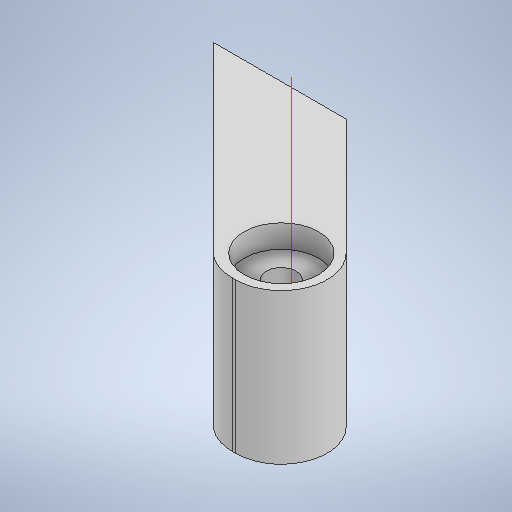
# Autodesk Inventor part: PingPongLauncherWinkel
Saved by Autodesk Inventor 2025 (Build 290162010, 162A)
## iProperties
Created: 2024-10-07
Part Number: PingPongLauncherWinkel
Material: Generisch
Document SubType Name: Modeling
Designer: max-h
Density: 1 g/cm^3
Appearance: Vorgabe
Author: max-h
Autodesk Inventor part; units mm, degrees
ref_plane "YZ Plane" through (0, 0, 0) normal (1, 0, 0) x (0, 1, 0)
ref_plane "XZ Plane" through (0, 0, 0) normal (0, 1, 0) x (-1, 0, 0)
ref_plane "XY Plane" through (0, 0, 0) normal (0, 0, 1) x (1, 0, 0)
sketch "Skizze1" plane through (0, 0, 0) normal (0, 1, 0) x (-1, 0, 0)
  line L0 (29, 0) -> (-13.4264, 42.4264)
  line L1 (0, 0) -> (29, 0)
  line L2 (-56.7117, 0) -> (43.2853, 0) projected
  line L3 (0, 0) -> (-42.4264, 42.4264)
  line L4 (-42.4264, 42.4264) -> (-13.4264, 42.4264)
  dimension "d0" = 60
  dimension "d1" = 45
  dimension "d99" = 29
  constraints: 8 end point, 2 parallel, 1 coincident, 1 point on line
  measures "d0" distance of L0.start L0.end
  measures "d1" angle of L0 L1
  measures "d99" distance of L1.start L0.start
extrude "Extrusion1" add sketch "Skizze1" along normal blind 32.8
ref_plane "Arbeitsebene1" through (21.9117, 0, 33.9411) normal (-0.7071068, 0, 0.7071068) x (0.7071068, 0, 0.7071068)
sketch "Skizze2" plane through (13.4264, 0, 42.4264) normal (-0.7071068, 0, 0.7071068) x (0.7071068, 0, 0.7071068)
  circle A0 centre (-31, 9.15) radius 2.125
  circle A1 centre (-49, 16.4) radius 2.125
  circle A2 centre (-31, 23.65) radius 2.125
  line L0 (0, 0) -> (0, 32.8) projected
  line L1 (-31, 9.15) -> (-31, 23.65) construction
  line L2 (-31, 23.65) -> (-49, 16.4) construction
  line L3 (-49, 16.4) -> (-31, 9.15) construction
  line L4 (-60, 0) -> (0, 0) construction
  line L5 (0, 16.4) -> (-60, 16.4) construction
  line L6 (-60, 0) -> (-60, 32.8) construction
  point P0 (-39.4939, 0)
  dimension "d5" = 4.25
  dimension "d7" = 32.8
  dimension "d8" = 14.5
  dimension "d10" = 18
  dimension "d89" = 11
  constraints: 8 end point, 3 centre point, 2 coincident, 2 equal radius, 2 midpoint, 1 horizontal, 1 point on line, 1 symmetric about line, 1 vertical
  measures "d5" diameter of A1
  measures "d7" diameter of L4 L5
  measures "d8" distance of L1.start L1.end
  measures "d10" distance from line of L1 A1.centre
  measures "d89" distance from line of L6 A1.centre
extrude "Extrusion2" cut sketch "Skizze2" against normal blind 50
sketch "Skizze7" plane through (21.9117, 0, 33.9411) normal (-0.7071068, 0, 0.7071068) x (0.7071068, 0, 0.7071068)
  circle A0 centre (-31, 9.15) radius 4.375
  circle A1 centre (-31, 23.65) radius 4.375
  circle A2 centre (-31, 9.15) radius 2.125 projected
  circle A3 centre (-31, 23.65) radius 2.125 projected
  circle A4 centre (-49, 16.4) radius 4.375
  circle A5 centre (-49, 16.4) radius 2.125 projected
  point P0 (-39.4939, 0)
  point P1 (-21, 9.15)
  point P2 (-17, 23.65)
  dimension "d39" = 8.75
  constraints: 3 centre point, 3 coincident, 2 equal radius
  measures "d39" diameter of A0
extrude "Extrusion7" cut sketch "Skizze7" along normal blind 0.5 and the other way blind 20 contours A0 | A1 | A2 | A3 | A4
sketch "Skizze8" plane through (21.9117, 0, 33.9411) normal (-0.7071068, 0, 0.7071068) x (0.7071068, 0, 0.7071068)
  circle A0 centre (-49, 16.4) radius 4.375
  circle A1 centre (-31, 9.15) radius 4.375 projected
  arc A2 (-48.5, 18.4653) -> (-48.5, 14.3347) centre (-49, 16.4) ccw projected
  point P0 (-39.4939, 0)
  point P1 (-41.5, 16.4)
  point P2 (-20.1844, 6.15)
  point P3 (-25.175, 7.8423)
  point P4 (-25.175, 10.4577)
  point P5 (-41.5, 16.4)
  constraints: 1 centre point, 1 coincident, 2 other
extrude "Extrusion8" add sketch "Skizze8" along normal blind 9 contours A0
fillet "Rundung2" radius 10 2 edges at (42.4264, 16.4, 42.4264) (13.4264, 16.4, 42.4264)
sketch "Skizze18" plane through (-12.7365, 16.4, -0.7071) normal (0.7071068, 0, -0.7071068) x (0, -1, 0)
  circle A0 centre (0, 0) radius 2.125 projected
  point P0 (16.4, -9.5061)
  point P1 (1.3077, -4.175)
  point P2 (-1.3077, -4.175)
  constraints: 1 other
extrude "Extrusion17" cut sketch "Skizze18" against normal blind 10
sketch "Skizze17" plane through (0, 0, 0) normal (0, -1, 0) x (1, 0, 0)
  circle A0 centre (18.2843, 32.4264) radius 8.125
  line L0 (13.4264, 42.4264) -> (18.2843, 42.4264) projected
  line L1 (25.3553, 25.3553) -> (0, 0) projected
  dimension "d85" = 16.25
  dimension "d86" = 10
  dimension "d87" = 10
  constraints: 1 centre point
  measures "d85" diameter of A0
  measures "d86" distance from line of L0 A0.centre
  measures "d87" distance from line of L1 A0.centre
extrude "Extrusion18" cut sketch "Skizze17" against normal blind 5
sketch "Skizze19" plane through (0, 32.8, 0) normal (0, 1, 0) x (1, 0, 0)
  circle A0 centre (18.2843, -32.4264) radius 8.125 projected
  point P0 (0, 0)
  point P1 (7.3738, -32.3738)
  point P2 (4.1947, -29.1947)
  constraints: 1 other
extrude "Extrusion19" cut sketch "Skizze19" against normal blind 5
sketch "Skizze20" plane through (18.2843, 5, 32.4264) normal (0, -1, 0) x (1, 0, 0)
  circle A0 centre (0, 0) radius 3.25
  circle A1 centre (0, 0) radius 8.125 projected
  point P0 (-18.2843, -32.4264)
  point P1 (2.248, -7.6777)
  point P2 (-2.248, -7.6777)
  dimension "d96" = 6.5
  constraints: 1 centre point, 1 coincident, 1 other
  measures "d96" diameter of A0
extrude "Extrusion20" cut sketch "Skizze20" against normal through all contours A0
